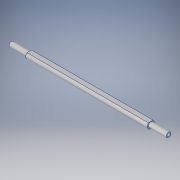
# Autodesk Inventor part: Storage Axle
Saved by Autodesk Inventor 2019.4 (Build 234330000, 330)
## iProperties
Created: 2020-01-27
Part Number: Storage Axle
Material: Aluminum 6061
Document SubType Name: Modeling
Designer: admin
Density: 2.7 g/cm^3
Appearance: Aluminum - Flat
Author: admin
Autodesk Inventor part; units mm, degrees
ref_plane "YZ Plane" through (0, 0, 0) normal (1, 0, 0) x (0, 1, 0)
ref_plane "XZ Plane" through (0, 0, 0) normal (0, 1, 0) x (-1, 0, 0)
ref_plane "XY Plane" through (0, 0, 0) normal (0, 0, 1) x (1, 0, 0)
sketch "Sketch1" plane through (0, 0, 0) normal (0, 0, 1) x (1, 0, 0)
  line L0 (0, 0) -> (0, 4)
  line L1 (0, 4) -> (30, 4)
  line L2 (30, 4) -> (30, 6)
  line L3 (30, 6) -> (234.6, 6)
  line L4 (234.6, 6) -> (234.6, 4)
  line L5 (234.6, 4) -> (264.6, 4)
  line L6 (264.6, 4) -> (264.6, 0)
  line L7 (264.6, 0) -> (0, 0)
  dimension "d0" = 4
  dimension "d1" = 6
  dimension "d2" = 204.6
  dimension "d3" = 30
  dimension "d4" = 30
  constraints: 16 end point, 6 perpendicular, 2 point on line, 1 vertical
  measures "d0" distance between parallel lines of L7 L1
  measures "d1" distance between parallel lines of L7 L3
  measures "d2" distance of L2.end L3.end
  measures "d3" distance of L4.end L5.end
  measures "d4" distance of L0.end L1.end
revolve "Revolution1" add sketch "Sketch1" angle 360 about axis through (264.6, 0, 0) along (-1, 0, 0)
sketch "Sketch2" plane through (234.6, 0, 0) normal (1, 0, 0) x (0, 0, -1)
  line L0 (-3.9686, 4.5) -> (3.9686, 4.5)
  circle A0 centre (0, 0) radius 6 projected
  dimension "d6" = 4.5
  constraints: 2 end point, 2 point on circle, 1 horizontal
  measures "d6" distance from line of A0.centre L0
extrude "Extrusion1" cut sketch "Sketch2" against normal through all contours A0 L0 picked at (0, 5)
sketch "Sketch3" plane through (264.6, 0, 0) normal (1, 0, 0) x (0, 0, -1)
  circle A0 centre (0, 0) radius 4 projected
  constraints: 1 coincident
hole "Hole1" at (264.6, 0, 0) direction (-1, 0, 0) diameter 5 end through all
body "Solid1"
